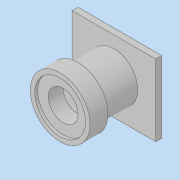
# Autodesk Inventor part: Camera
Saved by Autodesk Inventor 2017 (Build 210142000, 142)
## iProperties
Created: 2018-02-22
Part Number: Camera
Material: Generic
Document SubType Name: Modeling
Designer: Derek Wider
Density: 1 g/cm^3
Appearance: Default
Author: Derek Wider
Autodesk Inventor part; units mm, degrees
ref_plane "YZ Plane" through (0, 0, 0) normal (1, 0, 0) x (0, 1, 0)
ref_plane "XZ Plane" through (0, 0, 0) normal (0, 1, 0) x (-1, 0, 0)
ref_plane "XY Plane" through (0, 0, 0) normal (0, 0, 1) x (1, 0, 0)
sketch "Sketch1" plane through (0, 0, 0) normal (0, 0, 1) x (1, 0, 0)
  line L0 (0, 0) -> (14, 0)
  line L1 (14, 0) -> (14, 12)
  line L2 (14, 12) -> (0, 12)
  line L3 (0, 12) -> (0, 0)
  dimension "d0" = 14
  dimension "d1" = 12
  constraints: 8 end point, 2 parallel, 1 horizontal, 1 perpendicular
  measures "d0" distance of L0.start L0.end
  measures "d1" distance of L0.end L1.end
extrude "Extrusion1" add sketch "Sketch1" along normal blind 1
sketch "Sketch2" plane through (0, 0, 1) normal (0, 0, 1) x (1, 0, 0)
  line L0 (0, 0) -> (14, 0) construction
  line L1 (14, 0) -> (14, 12) construction
  line L2 (14, 12) -> (0, 12) construction
  line L3 (0, 12) -> (0, 0) construction
  circle A0 centre (7, 6) radius 4
  dimension "d4" = 8
  constraints: 1 centre point
  measures "d4" diameter of A0
extrude "Extrusion2" add sketch "Sketch2" along normal blind 6
sketch "Sketch3" plane through (7, 6, 7) normal (0, 0, 1) x (1, 0, 0)
  circle A0 centre (0, 0) radius 5
  circle A1 centre (0, 0) radius 3
  circle A2 centre (0, 0) radius 4
  point P0 (-7, -6)
  dimension "d7" = 10
  dimension "d8" = 6
  constraints: 3 centre point, 2 coincident
  measures "d7" diameter of A0
  measures "d8" diameter of A1
extrude "Extrusion3" add sketch "Sketch3" along normal blind 3 contours A0 | A1 | A2
sketch "Sketch4" plane through (7, 6, 10) normal (0, 0, 1) x (1, 0, 0)
  circle A0 centre (0, 0) radius 2.5
  circle A1 centre (0, 0) radius 4.25
  circle A2 centre (0, 0) radius 5 projected
  point P0 (-7, -6)
  dimension "d11" = 5
  dimension "d12" = 8.5
  constraints: 2 centre point, 1 coincident
  measures "d11" diameter of A0
  measures "d12" diameter of A1
extrude "Extrusion4" cut sketch "Sketch4" against normal blind 3 contours A0
extrude "Extrusion5" cut sketch "Sketch4" against normal blind 0.5 contours A1
body "Solid1"
